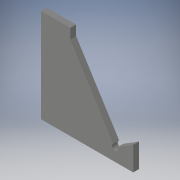
# Autodesk Inventor part: JIG1
Saved by Autodesk Inventor 2018 (Build 220112000, 112)
## iProperties
Created: 2018-11-15
Part Number: JIG1
Material: A36
Document SubType Name: Sheet Metal
Designer: S.O.
Stock Number: =<Thickness> - <Material>
Density: 7.80573 g/cm^3
Sheet Metal Rule: Default
Appearance: A36
Author: S.O.
Thickness: 0.500 in
Autodesk Inventor part; units mm, degrees
ref_plane "Right" through (0, 0, 0) normal (1, 0, 0) x (0, 1, 0)
ref_plane "Top" through (0, 0, 0) normal (0, 1, 0) x (-1, 0, 0)
ref_plane "Front" through (0, 0, 0) normal (0, 0, 1) x (1, 0, 0)
sketch "Sketch1" plane through (0, 0, 0) normal (0, 0, 1) x (1, 0, 0)
  line L0 (0, 0) -> (-200, 0) construction
  line L1 (-200, 0) -> (-200, 400) construction
  line L2 (-200, 400) -> (0, 400) construction
  line L3 (0, 400) -> (0, 0) construction
  line L4 (11.905, 82.55) -> (10, 82.55)
  line L5 (10, 82.55) -> (10, 50.8)
  line L6 (10, 50.8) -> (11.905, 50.8)
  line L7 (11.905, 50.8) -> (11.905, 82.55)
  line L8 (-46.4241, 188.377) -> (10, 98.0795) construction
  line L9 (10, 98.0795) -> (10, 57.975) construction
  line L10 (10, 57.975) -> (-21.8066, 38.1) construction
  line L11 (-21.8066, 38.1) -> (-57.8523, 55.6807) construction
  line L12 (-57.8523, 55.6807) -> (-114.2764, 145.9781) construction
  line L13 (-114.2764, 145.9781) -> (-46.4241, 188.377) construction
  line L14 (0, 51.7263) -> (0, 0)
  line L15 (0, 0) -> (-200, 0)
  line L16 (-200, 0) -> (-200, 203.2)
  line L17 (-200, 203.2) -> (-136.5, 203.2)
  line L18 (0, 51.7263) -> (-34.4444, 30.203)
  line L19 (-43.1944, 32.2232) -> (-136.5, 181.5433)
  line L20 (-136.5, 181.5433) -> (-136.5, 203.2)
  arc A0 (-43.1944, 32.2232) -> (-34.4444, 30.203) centre (-39.8295, 26.8381) ccw
  dimension "d0" = 200
  dimension "d1" = 400
  dimension "d2" = 1.905
  dimension "d3" = 31.75
  dimension "d4" = 10
  dimension "d5" = 50.8
  dimension "d6" = 32
  dimension "d7" = 32
  dimension "d8" = 80.01
  dimension "d9" = 34.0106
  dimension "d10" = 140.4874
  dimension "d11" = 38.1
  dimension "d12" = 63.5
  dimension "d13" = 203.2
  dimension "d14" = 12.7
  dimension "d15" = 52.3469
  dimension "d16" = 55.7119
  measures "d0" distance of L1.end L2.end
  measures "d1" distance of L2.end L0.start
  measures "d2" distance of L4.start L4.end
  measures "d3" distance of L6.end L4.start
  measures "d4" distance between parallel lines of L5 L3
  measures "d5" distance from line of L6.end L0
  measures "d6" angle of L11 L12
  measures "d7" angle of L9 L8
  measures "d8" distance between parallel lines of L12 L8
  measures "d9" distance from line of L8.end L10
  measures "d10" distance between parallel lines of L13 L10
  measures "d11" distance from line of L0 L10.end
  measures "d12" distance of L16.end L17.end
  measures "d13" distance between parallel lines of L0 L17
  measures "d14" diameter of A0
  measures "d15" distance from line of L18.end L4
  measures "d16" distance from line of A0.centre L4
extrude "Plate1" add sketch "Sketch1" along normal blind 12.7 contours L14 L15 L16 L17 L20 L19 A0 L18
equation "\"d7\" = d6"
equation "\"d17\" = Thickness"
equation "\"BendRadius\" = Thickness"
equation "\"BendReliefWidth\" = 0.5 * Thickness"
equation "\"BendReliefDepth\" = 0.5 * Thickness"
equation "\"CornerReliefSize\" = 4 * Thickness"
equation "\"MinimumRemnant\" = 2 * Thickness"
equation "\"TransitionRadius\" = BendRadius"
equation "\"JacobiRadiusSize\" = BendRadius"
equation "\"Thickness\" = 12.7"
body "Solid1"
